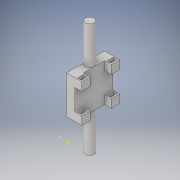
# Autodesk Inventor part: Spiegelhalter2.0
Saved by Autodesk Inventor 2017 (Build 210142000, 142)
## iProperties
Part Number: Spiegelhalter2.0
Material: Generisch
Document SubType Name: Modeling
Designer: pgmadmin
Density: 1 g/cm^3
Appearance: Vorgabe
Author: pgmadmin
Autodesk Inventor part; units mm, degrees
ref_plane "YZ Plane" through (0, 0, 0) normal (1, 0, 0) x (0, 1, 0)
ref_plane "XZ Plane" through (0, 0, 0) normal (0, 1, 0) x (-1, 0, 0)
ref_plane "XY Plane" through (0, 0, 0) normal (0, 0, 1) x (1, 0, 0)
sketch "Skizze1" plane through (0, 0, 0) normal (1, 0, 0) x (0, 1, 0)
  line L0 (52.3929, 62.5179) -> (7.3929, 62.5179)
  line L1 (7.3929, 62.5179) -> (7.3929, 17.5179)
  line L2 (7.3929, 17.5179) -> (52.3929, 17.5179)
  line L3 (52.3929, 17.5179) -> (52.3929, 62.5179)
  point P0 (0, 0)
  dimension "d0" = 45
  dimension "d1" = 45
  constraints: 8 end point, 2 parallel, 1 horizontal, 1 perpendicular
  measures "d0" distance of L1.end L2.end
  measures "d1" distance of L0.end L1.end
extrude "Extrusion1" add sketch "Skizze1" along normal blind 10
sketch "Skizze2" plane through (0, 7.3929, 62.5179) normal (0, 0, 1) x (1, 0, 0)
  line L0 (0, 0) -> (10, 0) projected
  line L1 (0, 45) -> (0, 0) projected
  line L2 (10, 45) -> (10, 0) projected
  circle A0 centre (5, 22.5) radius 5
  point P0 (0, -7.3929)
  dimension "d4" = 22.5
  dimension "d7" = 10
  dimension "d18" = 5
  constraints: 1 centre point, 1 coincident
  measures "d4" distance from line of L0 point (5, 22.5)
  measures "d7" diameter of A0
  measures "d18" distance from line of L1 point (5, 22.5)
extrude "Extrusion2" add sketch "Skizze2" along normal blind 45 contours A0
sketch "Skizze3" plane through (0, 7.3929, 17.5179) normal (0, 0, -1) x (-1, 0, 0)
  line L0 (0, 45) -> (-10, 45) projected
  circle A0 centre (-5, 22.5) radius 5
  line L1 (0, 0) -> (0, 45) projected
  point P0 (0, -7.3929)
  dimension "d10" = 22.5
  dimension "d11" = 10
  dimension "d19" = 5
  constraints: 1 centre point, 1 coincident
  measures "d10" distance from line of L0 point (-5, 22.5)
  measures "d11" diameter of A0
  measures "d19" distance from line of L1 A0.centre
extrude "Extrusion3" add sketch "Skizze3" along normal blind 45
sketch "Skizze4" plane through (10, 0, 0) normal (1, 0, 0) x (0, 0, -1)
  point P0 (0, 0)
sketch "Skizze6" plane through (10, 52.3929, 59.5179) normal (1, 0, 0) x (0, 0, -1)
  point P0 (59.5179, -52.3929)
sketch "Skizze7" plane through (10, 52.3929, 59.5179) normal (1, 0, 0) x (0, 0, -1)
  point P0 (59.5179, -52.3929)
sketch "Skizze10" plane through (10, 0, 0) normal (1, 0, 0) x (0, 0, -1)
  line L0 (-62.5179, 29.8929) -> (-62.5179, 7.3929) projected
  line L1 (-62.5179, 52.3929) -> (-62.5179, 29.8929) projected
  line L2 (-17.5179, 52.3929) -> (-62.5179, 52.3929) projected
  line L3 (-17.5179, 29.8929) -> (-17.5179, 52.3929) projected
  line L4 (-17.5179, 24.8929) -> (27.4821, 24.8929) projected
  line L5 (-17.5179, 7.3929) -> (-17.5179, 29.8929) projected
  line L6 (-62.5179, 7.3929) -> (-17.5179, 7.3929) projected
  line L7 (-62.5179, 7.3929) -> (-52.5179, 7.3929)
  line L8 (-52.5179, 7.3929) -> (-52.5179, 17.3929)
  line L9 (-52.5179, 17.3929) -> (-62.5179, 17.3929)
  line L10 (-62.5179, 17.3929) -> (-62.5179, 7.3929)
  line L11 (-62.5179, 52.3929) -> (-52.5179, 52.3929)
  line L12 (-52.5179, 52.3929) -> (-52.5179, 42.3929)
  line L13 (-52.5179, 42.3929) -> (-62.5179, 42.3929)
  line L14 (-62.5179, 42.3929) -> (-62.5179, 52.3929)
  line L15 (-17.5179, 7.3929) -> (-17.5179, 29.8929) projected
  line L16 (-17.5179, 7.3929) -> (-27.5179, 7.3929)
  line L17 (-27.5179, 7.3929) -> (-27.5179, 17.3929)
  line L18 (-27.5179, 17.3929) -> (-17.5179, 17.3929)
  line L19 (-17.5179, 17.3929) -> (-17.5179, 7.3929)
  line L20 (-17.5179, 52.3929) -> (-27.5179, 52.3929)
  line L21 (-27.5179, 52.3929) -> (-27.5179, 42.3929)
  line L22 (-27.5179, 42.3929) -> (-17.5179, 42.3929)
  line L23 (-17.5179, 42.3929) -> (-17.5179, 52.3929)
  point P0 (0, 0)
  dimension "d46" = 10
  dimension "d47" = 10
  dimension "d48" = 10
  dimension "d49" = 10
  dimension "d50" = 10
  dimension "d51" = 10
  dimension "d52" = 10
  dimension "d53" = 10
  constraints: 32 end point, 8 parallel, 4 horizontal, 4 perpendicular
  measures "d46" distance of L9.end L8.end
  measures "d47" distance of L8.end L7.end
  measures "d48" distance of L12.end L13.end
  measures "d49" distance of L11.end L12.end
  measures "d50" distance of L17.end L18.end
  measures "d51" distance of L16.end L17.end
  measures "d52" distance of L22.end L21.end
  measures "d53" distance of L21.end L20.end
extrude "Extrusion5" add sketch "Skizze10" along normal blind 8 contours L9 L8 L6 L0 | L1 L2 L12 L13 | L17 L18 L5 L6 | L2 L3 L22 L21
sketch "Skizze11" plane through (0, 29.8929, 62.5179) normal (0, 0, 1) x (1, 0, 0)
  line L0 (11.75, 13.85) -> (16.25, 13.85)
  line L1 (16.25, 13.85) -> (16.25, 21.15)
  line L2 (16.25, 21.15) -> (11.75, 21.15)
  line L3 (11.75, 21.15) -> (11.75, 13.85)
  line L4 (11.75, -21.15) -> (16.25, -21.15)
  line L5 (16.25, -21.15) -> (16.25, -13.85)
  line L6 (16.25, -13.85) -> (11.75, -13.85)
  line L7 (11.75, -13.85) -> (11.75, -21.15)
  line L8 (0, -22.5) -> (18, -22.5) projected
  line L9 (10, 12.5) -> (18, 12.5) projected
  line L10 (18, 22.5) -> (18, 12.5) projected
  point P0 (0, -29.8929)
  dimension "d56" = 4.5
  dimension "d57" = 7.3
  dimension "d58" = 4.5
  dimension "d59" = 7.3
  dimension "d60" = 1.35
  dimension "d61" = 1.35
  dimension "d62" = 1.75
  constraints: 16 end point, 4 parallel, 2 horizontal, 2 perpendicular, 1 point on line
  measures "d56" distance of L2.end L1.end
  measures "d57" distance of L1.end L0.end
  measures "d58" distance of L6.end L5.end
  measures "d59" distance of L5.end L4.end
  measures "d60" distance between parallel lines of L8 L4
  measures "d61" distance between parallel lines of L9 L0
  measures "d62" distance between parallel lines of L10 L1
extrude "Extrusion6" cut sketch "Skizze11" against normal blind 8
sketch "Skizze12" plane through (10, 7.3929, 27.5179) normal (0, 0, 1) x (1, 0, 0)
  line L0 (1.75, 1.35) -> (6.25, 1.35)
  line L1 (6.25, 1.35) -> (6.25, 8.65)
  line L2 (6.25, 8.65) -> (1.75, 8.65)
  line L3 (1.75, 8.65) -> (1.75, 1.35)
  line L4 (1.75, 36.35) -> (6.25, 36.35)
  line L5 (6.25, 36.35) -> (6.25, 43.65)
  line L6 (6.25, 43.65) -> (1.75, 43.65)
  line L7 (1.75, 43.65) -> (1.75, 36.35)
  line L8 (8, 10) -> (8, 0) projected
  line L9 (0, 0) -> (8, 0) projected
  line L10 (0, 35) -> (8, 35) projected
  point P0 (-10, -7.3929)
  dimension "d65" = 1.75
  dimension "d66" = 1.35
  dimension "d67" = 7.3
  dimension "d68" = 4.5
  dimension "d69" = 7.3
  dimension "d70" = 4.5
  dimension "d71" = 1.35
  constraints: 16 end point, 4 parallel, 2 horizontal, 2 perpendicular, 1 point on line
  measures "d65" distance between parallel lines of L1 L8
  measures "d66" distance between parallel lines of L9 L0
  measures "d67" distance between parallel lines of L2 L0
  measures "d68" distance between parallel lines of L3 L1
  measures "d69" distance of L6.end L4.start
  measures "d70" distance of L4.start L4.end
  measures "d71" distance between parallel lines of L10 L4
extrude "Extrusion7" cut sketch "Skizze12" against normal blind 8
sketch "Skizze13" plane through (0, 0, 0) normal (-1, 0, 0) x (0, 0, 1)
  line L0 (62.5179, 52.3929) -> (62.5179, 29.8929) projected
  line L1 (17.5179, 52.3929) -> (62.5179, 52.3929) projected
  line L2 (62.5179, 29.8929) -> (62.5179, 7.3929) projected
  line L3 (62.5179, 7.3929) -> (17.5179, 7.3929) projected
  line L4 (17.5179, 7.3929) -> (17.5179, 29.8929) projected
  line L5 (17.5179, 29.8929) -> (17.5179, 52.3929) projected
  circle A0 centre (57.5179, 47.3929) radius 2
  circle A1 centre (57.5179, 12.3929) radius 2
  circle A2 centre (22.5179, 47.3929) radius 2
  circle A3 centre (22.5179, 12.3929) radius 2
  point P0 (0, 0)
  dimension "d74" = 5
  dimension "d75" = 5
  dimension "d76" = 5
  dimension "d77" = 5
  dimension "d78" = 5
  dimension "d79" = 5
  dimension "d80" = 5
  dimension "d81" = 5
  dimension "d82" = 4
  dimension "d83" = 4
  dimension "d84" = 4
  dimension "d85" = 4
  constraints: 4 centre point, 4 coincident
  measures "d74" distance from line of L0 point (57.518, 47.393)
  measures "d75" distance from line of L1 point (57.518, 47.393)
  measures "d76" distance from line of L2 point (57.518, 12.393)
  measures "d77" distance from line of L3 point (57.518, 12.393)
  measures "d78" distance from line of L3 point (22.518, 12.393)
  measures "d79" distance from line of L4 point (22.518, 12.393)
  measures "d80" distance from line of L5 point (22.518, 47.393)
  measures "d81" distance from line of L1 point (22.518, 47.393)
  measures "d82" diameter of A0
  measures "d83" diameter of A1
  measures "d84" diameter of A2
  measures "d85" diameter of A3
extrude "Extrusion8" cut sketch "Skizze13" against normal blind 12 contours A0 | A1 | A2 | A3
sketch "Skizze14" plane through (0, 0, 0) normal (-1, 0, 0) x (0, 0, 1)
  point P0 (0, 0)
sketch "Skizze15" plane through (10, 0, 0) normal (1, 0, 0) x (0, 0, -1)
  point P0 (0, 0)
